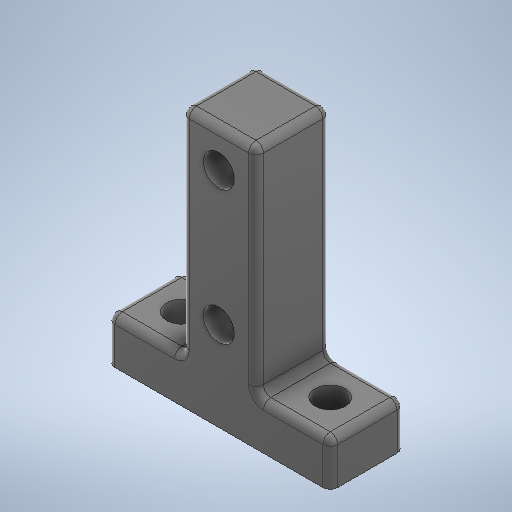
# Autodesk Inventor part: al_rod_bracket
Saved by Autodesk Inventor 2026.2 (Build 302298010, 298A)
## iProperties
Created: 2026-04-12
Part Number: al_rod_bracket
Material: ABS Plastic
Document SubType Name: Modeling
Designer: chris
Density: 1.06 g/cm^3
Appearance: Smooth - White
Author: chris
Autodesk Inventor part; units mm, degrees
ref_plane "YZ Plane" through (0, 0, 0) normal (1, 0, 0) x (0, 1, 0)
ref_plane "XZ Plane" through (0, 0, 0) normal (0, 1, 0) x (-1, 0, 0)
ref_plane "XY Plane" through (0, 0, 0) normal (0, 0, 1) x (1, 0, 0)
sketch "Sketch1" plane through (0, 0, 0) normal (0, 1, 0) x (-1, 0, 0)
  line L0 (15, 7.5) -> (-15, 7.5)
  line L1 (-15, 7.5) -> (-15, -7.5)
  line L2 (-15, -7.5) -> (15, -7.5)
  line L3 (15, -7.5) -> (15, 7.5)
  line L4 (15, 7.5) -> (-15, -7.5) construction
  line L5 (-15, 7.5) -> (15, -7.5) construction
  point P0 (0, 0)
  dimension "d0" = 30
  dimension "d1" = 15
  constraints: 12 end point, 2 midpoint, 2 parallel, 1 horizontal, 1 perpendicular
  measures "d0" distance of L2.end L1.end
  measures "d1" distance of L1.end L0.end
extrude "Extrusion1" add sketch "Sketch1" along normal blind 5
sketch "Sketch2" plane through (0, 5, 0) normal (0, 1, 0) x (1, 0, 0)
  line L0 (5, -7.5) -> (-5, -7.5)
  line L1 (-5, -7.5) -> (-5, 7.5)
  line L2 (-5, 7.5) -> (5, 7.5)
  line L3 (5, 7.5) -> (5, -7.5)
  line L4 (5, -7.5) -> (-5, 7.5) construction
  line L5 (-5, -7.5) -> (5, 7.5) construction
  point P0 (0, 0)
  dimension "d4" = 10
  dimension "d5" = 15
  constraints: 12 end point, 2 midpoint, 2 parallel, 1 horizontal, 1 perpendicular
  measures "d4" distance of L1.end L2.end
  measures "d5" distance of L0.end L1.end
extrude "Extrusion2" add sketch "Sketch2" along normal blind 30
sketch "Sketch3" plane through (-15, 0, 7.5) normal (0, 0, 1) x (1, 0, 0)
  circle A0 centre (15, 12) radius 2.1
  line L0 (0, 0) -> (30, 0) projected
  point P0 (15, 0)
  dimension "d8" = 4.2
  dimension "d9" = 12
  constraints: 1 centre point
  measures "d8" diameter of A0
  measures "d9" distance from line of L0 A0.centre
extrude "Extrusion3" cut sketch "Sketch3" against normal blind 10
sketch "Sketch4" plane through (0, 5, 0) normal (0, 1, 0) x (1, 0, 0)
  circle A0 centre (-10, 2.5) radius 2.05
  line L0 (-15, 7.5) -> (-15, -7.5) projected
  line L1 (15, 7.5) -> (-15, 7.5) projected
  circle A1 centre (10, 2.5) radius 2.05
  line L2 (15, -7.5) -> (15, 7.5) projected
  line L3 (15, 7.5) -> (-15, 7.5) projected
  point P0 (0, 0)
  point P1 (-5, 7.5)
  point P2 (-10, 7.5)
  point P3 (5, 7.5)
  dimension "d12" = 4.1
  dimension "d13" = 5
  dimension "d14" = 5
  dimension "d15" = 4.1
  dimension "d16" = 5
  dimension "d17" = 5
  constraints: 2 centre point, 1 point on line
  measures "d12" diameter of A0
  measures "d13" distance from line of L0 A0.centre
  measures "d14" distance of point (-10, 7.5) A0.centre
  measures "d15" diameter of A1
  measures "d16" distance from line of L2 A1.centre
  measures "d17" distance from line of L3 A1.centre
extrude "Extrusion4" cut sketch "Sketch4" against normal through all
sketch "Sketch5" plane through (-15, 0, 7.5) normal (0, 0, 1) x (1, 0, 0)
  circle A0 centre (15, 30) radius 2.1
  line L0 (10, 35) -> (20, 35) projected
  point P0 (15, 0)
  dimension "d20" = 4.2
  dimension "d21" = 5
  constraints: 1 centre point
  measures "d20" diameter of A0
  measures "d21" distance from line of L0 A0.centre
extrude "Extrusion5" cut sketch "Sketch5" against normal blind 10
sketch "Sketch8" plane through (-15, 0, 7.5) normal (0, 0, 1) x (1, 0, 0)
  circle A0 centre (15, 30) radius 2.1 projected
  circle A1 centre (15, 12) radius 2.1 projected
  circle A2 centre (15, 30) radius 2.1
  circle A3 centre (15, 12) radius 2.1
  circle A4 centre (15, 30) radius 2.1 projected
  circle A5 centre (15, 12) radius 2.1 projected
  line L0 (0, 0) -> (30, 0) projected
  line L1 (30, 0) -> (30, 5) projected
  line L2 (20, 5) -> (30, 5) projected
  line L3 (20, 5) -> (20, 35) projected
  line L4 (10, 35) -> (20, 35) projected
  line L5 (10, 5) -> (10, 35) projected
  line L6 (0, 5) -> (10, 5) projected
  line L7 (0, 0) -> (0, 5) projected
  line L8 (10, 35) -> (10, 5)
  line L9 (0, 5) -> (0, 0)
  line L10 (30, 0) -> (30, 5)
  line L11 (20, 5) -> (20, 35)
  point P0 (15, 0)
  constraints: 8 end point, 2 centre point, 2 coincident, 2 collinear, 2 concentric, 1 parallel, 1 vertical
extrude "Extrusion7" cut sketch "Sketch8" against normal blind 5
sketch "Sketch9" plane through (0, 5, 0) normal (0, 1, 0) x (1, 0, 0)
  line L0 (-15, -2.5) -> (-5, -2.5) projected
  line L1 (-5, -2.5) -> (-5, 7.5) projected
  line L2 (-5, 7.5) -> (-15, 7.5) projected
  line L3 (-15, 7.5) -> (-15, -2.5) projected
  circle A0 centre (-10, 2.5) radius 2.05 projected
  line L4 (5, -2.5) -> (15, -2.5) projected
  line L5 (15, -2.5) -> (15, 7.5) projected
  line L6 (15, 7.5) -> (5, 7.5) projected
  line L7 (5, 7.5) -> (5, -2.5) projected
  circle A1 centre (10, 2.5) radius 2.05 projected
  point P0 (0, 0)
extrude "Extrusion8" add sketch "Sketch9" along normal blind 1
fillet "Fillet1" radius 1 20 edges at (0, 35, 2.5) (5, 35, -2.5) (0, 35, -7.5) (-5, 35, -2.5) (5, 20.5, 2.5) (5, 20.5, -7.5) (-5, 20.5, 2.5) (-5, 20.5, -7.5) (5, 6, -2.5) (-5, 6, -2.5) (-15, 6, -2.5) (-10, 6, 2.5) (10, 6, 2.5) (15, 6, -2.5) (10, 6, -7.5) (-10, 6, -7.5) (15, 3, 2.5) (15, 3, -7.5) (-15, 3, 2.5) (-15, 3, -7.5)
body "Solid1"
